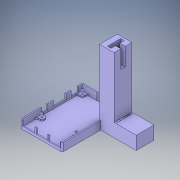
# Autodesk Inventor part: BaseStation.0027
Saved by Autodesk Inventor 2018 (Build 220112000, 112)
## iProperties
Material: Générique
Document SubType Name: Modeling
Density: 1 g/cm^3
Appearance: Par défaut(1)
Autodesk Inventor part; units mm, degrees
ref_plane "YZ Plane" through (0, 0, 0) normal (1, 0, 0) x (0, 1, 0)
ref_plane "XZ Plane" through (0, 0, 0) normal (0, 1, 0) x (-1, 0, 0)
ref_plane "XY Plane" through (0, 0, 0) normal (0, 0, 1) x (1, 0, 0)
sketch "Esquisse1" plane through (0, 0, 0) normal (0, 0, 1) x (1, 0, 0)
  line L0 (-30, -44.5) -> (30, -44.5)
  line L1 (30, -44.5) -> (30, 44.5)
  line L2 (30, 44.5) -> (-30, 44.5)
  line L3 (-30, 44.5) -> (-30, -44.5)
  line L4 (-30, -44.5) -> (30, 44.5) construction
  line L5 (30, -44.5) -> (-30, 44.5) construction
  point P0 (0, 0)
  dimension "Largeur_boite" = 60
  dimension "Longueur_boite" = 89
  constraints: 12 end point, 2 midpoint, 2 parallel, 1 horizontal, 1 perpendicular
  measures "Largeur_boite" distance of L2.end L1.end
  measures "Longueur_boite" distance of L1.end L0.end
extrude "Embase" add sketch "Esquisse1" along normal mid plane 11.5
shell "Coque" thickness 1.6 removed faces 1 at (-10, 14.8333, 5.75)
sketch "Esquisse2" plane through (-28.4, -42.9, -4.15) normal (0, 0, 1) x (1, 0, 0)
  line L0 (0, 85.8) -> (7.5, 85.8)
  line L1 (7.5, 85.8) -> (7.5, 78.3)
  line L2 (7.5, 78.3) -> (0, 78.3)
  line L3 (0, 78.3) -> (0, 85.8)
  line L4 (0, 85.8) -> (7.5, 78.3) construction
  line L5 (7.5, 85.8) -> (0, 78.3) construction
  line L6 (0, 27.8) -> (7.5, 27.8)
  line L7 (7.5, 27.8) -> (7.5, 20.3)
  line L8 (7.5, 20.3) -> (0, 20.3)
  line L9 (0, 20.3) -> (0, 27.8)
  line L10 (0, 27.8) -> (7.5, 20.3) construction
  line L11 (7.5, 27.8) -> (0, 20.3) construction
  line L12 (49.3, 85.8) -> (56.8, 85.8)
  line L13 (56.8, 85.8) -> (56.8, 78.3)
  line L14 (56.8, 78.3) -> (49.3, 78.3)
  line L15 (49.3, 78.3) -> (49.3, 85.8)
  line L16 (49.3, 85.8) -> (56.8, 78.3) construction
  line L17 (56.8, 85.8) -> (49.3, 78.3) construction
  line L18 (48.7, 27.8) -> (56.8, 27.8)
  line L19 (56.8, 27.8) -> (56.8, 20.3)
  line L20 (56.8, 20.3) -> (48.7, 20.3)
  line L21 (48.7, 20.3) -> (48.7, 27.8)
  line L22 (48.7, 27.8) -> (56.8, 20.3) construction
  line L23 (56.8, 27.8) -> (48.7, 20.3) construction
  line L24 (0, 85.8) -> (56.8, 85.8) projected
  line L25 (0, 0) -> (0, 85.8) projected
  line L26 (56.8, 85.8) -> (56.8, 0) projected
  point P0 (28.4, 42.9)
  point P1 (3.75, 82.05)
  point P2 (3.75, 24.05)
  point P3 (53.05, 82.05)
  point P4 (52.75, 24.05)
  point P5 (3.75, 24.05)
  point P6 (52.75, 24.05)
  point P7 (53.05, 82.05)
  point P8 (3.75, 82.05)
  dimension "d5" = 58
  dimension "d6" = 49
  dimension "Largeur_support" = 7.5
  dimension "d8" = 7.5
  dimension "d9" = 7.5
  dimension "d10" = 7.5
  constraints: 48 end point, 12 midpoint, 8 parallel, 5 collinear, 4 horizontal, 4 perpendicular, 4 point on line, 2 horizontal alignment
  measures "d5" vertical distance of point (53.05, 82.05) point (52.75, 24.05)
  measures "d6" distance of point (52.75, 24.05) point (3.75, 24.05)
  measures "Largeur_support" distance of L0.end L1.end
  measures "d8" distance of L1.end L2.end
  measures "d9" distance of L13.end L14.end
  measures "d10" distance between parallel lines of L8 L6
extrude "Support axe" add sketch "Esquisse2" along normal blind 2
sketch "Esquisse3" plane through (-28.4, -42.9, -2.15) normal (0, 0, 1) x (1, 0, 0)
  line L0 (49.3, 85.8) -> (56.8, 85.8) construction
  line L1 (49.3, 85.8) -> (49.3, 78.3) construction
  line L2 (49.3, 78.3) -> (56.8, 78.3) construction
  line L3 (56.8, 85.8) -> (56.8, 78.3) construction
  line L4 (0, 85.8) -> (7.5, 85.8) construction
  line L5 (0, 78.3) -> (0, 85.8) construction
  line L6 (0, 78.3) -> (7.5, 78.3) construction
  line L7 (7.5, 78.3) -> (7.5, 85.8) construction
  line L8 (7.5, 27.8) -> (0, 27.8) construction
  line L9 (0, 20.3) -> (0, 27.8) construction
  line L10 (0, 20.3) -> (7.5, 20.3) construction
  line L11 (7.5, 20.3) -> (7.5, 27.8) construction
  line L12 (56.8, 27.8) -> (48.7, 27.8) construction
  line L13 (48.7, 27.8) -> (48.7, 20.3) construction
  line L14 (48.7, 20.3) -> (56.8, 20.3) construction
  line L15 (56.8, 27.8) -> (56.8, 20.3) construction
  circle A0 centre (3.75, 82.05) radius 1.25
  circle A1 centre (52.75, 82.05) radius 1.25
  circle A2 centre (52.75, 24.05) radius 1.25
  circle A3 centre (3.75, 24.05) radius 1.25
  point P0 (28.4, 42.9)
  point P1 (7.5, 24.05)
  point P2 (48.7, 24.05)
  point P3 (7.5, 82.05)
  point P4 (49.3, 82.05)
  point P5 (3.75, 78.3)
  point P6 (53.05, 78.3)
  point P7 (3.75, 20.3)
  point P8 (52.75, 20.3)
  dimension "Hauteur_axe" = 2.5
  dimension "d14" = 2.5
  dimension "d15" = 2.5
  dimension "d16" = 2.5
  dimension "d54" = 3.45
  constraints: 8 midpoint, 4 centre point, 4 horizontal alignment, 3 vertical alignment
  measures "Hauteur_axe" diameter of A0
  measures "d14" diameter of A1
  measures "d15" diameter of A3
  measures "d16" diameter of A2
  measures "d54" distance from line of L1 A1.centre
extrude "Axe" add sketch "Esquisse3" along normal blind 7
sketch "Esquisse4" plane through (-30, -44.5, -5.75) normal (0, -1, 0) x (1, 0, 0)
  line L0 (3.5, 4) -> (21, 4)
  line L1 (21, 4) -> (21, 11.5)
  line L2 (21, 11.5) -> (3.5, 11.5)
  line L3 (3.5, 11.5) -> (3.5, 4)
  line L4 (23, 4) -> (39, 4)
  line L5 (39, 4) -> (39, 11.5)
  line L6 (39, 11.5) -> (23, 11.5)
  line L7 (23, 11.5) -> (23, 4)
  line L8 (41, 4) -> (57, 4)
  line L9 (57, 4) -> (57, 11.5)
  line L10 (57, 11.5) -> (41, 11.5)
  line L11 (41, 11.5) -> (41, 4)
  line L12 (0, 11.5) -> (0, 0) projected
  line L13 (0, 11.5) -> (60, 11.5) projected
  line L14 (60, 0) -> (0, 0) projected
  point P0 (30, 5.75)
  dimension "d19" = 17.5
  dimension "d20" = 16
  dimension "d21" = 16
  dimension "d22" = 3.5
  dimension "d23" = 2
  dimension "d24" = 2
  dimension "d28" = 4
  constraints: 24 end point, 6 parallel, 3 collinear, 3 horizontal, 3 perpendicular, 2 point on line
  measures "d19" distance of L1.end L2.end
  measures "d20" distance of L5.end L6.end
  measures "d21" distance of L9.end L10.end
  measures "d22" distance between parallel lines of L12 L3
  measures "d23" distance between parallel lines of L1 L7
  measures "d24" distance between parallel lines of L5 L11
  measures "d28" distance between parallel lines of L14 L0
extrude "Passage USB/Ethernet" cut sketch "Esquisse4" against normal up to surface (1.6 mm away)
sketch "Esquisse6" plane through (-30, -44.5, 5.75) normal (-1, 0, 0) x (0, 0, 1)
  line L0 (-7, 64) -> (0, 64)
  line L1 (0, 64) -> (0, 46)
  line L2 (0, 46) -> (-7, 46)
  line L3 (-7, 46) -> (-7, 64)
  line L4 (-11.5, 89) -> (0, 89) projected
  line L5 (0, 89) -> (0, 0) projected
  point P0 (-5.75, 44.5)
  dimension "d29" = 25
  dimension "d30" = 18
  dimension "profondeur_passage" = 7
  constraints: 8 end point, 2 parallel, 1 collinear, 1 horizontal, 1 perpendicular
  measures "d29" distance between parallel lines of L4 L0
  measures "d30" distance of L0.end L1.end
  measures "profondeur_passage" distance between parallel lines of L5 L3
extrude "Passage HDMI" cut sketch "Esquisse6" against normal up to surface (1.6 mm away)
sketch "Esquisse8" plane through (-30, -44.5, -5.75) normal (-1, 0, 0) x (0, 0, 1)
  line L0 (4.5, 81.5) -> (11.5, 81.5)
  line L1 (11.5, 81.5) -> (11.5, 71.5)
  line L2 (11.5, 71.5) -> (4.5, 71.5)
  line L3 (4.5, 71.5) -> (4.5, 81.5)
  line L4 (11.5, 89) -> (11.5, 64) projected
  line L5 (0, 89) -> (11.5, 89) projected
  point P0 (5.75, 44.5)
  dimension "d34" = 10
  dimension "d35" = 7
  dimension "d36" = 7.5
  constraints: 8 end point, 2 parallel, 1 collinear, 1 horizontal, 1 perpendicular
  measures "d34" distance of L0.end L1.end
  measures "d35" distance between parallel lines of L4 L3
  measures "d36" distance between parallel lines of L5 L0
extrude "Passage chargeur" cut sketch "Esquisse8" against normal up to surface (1.6 mm away)
sketch "Esquisse10" plane through (-30, 44.5, 5.75) normal (0, 1, 0) x (1, 0, 0)
  line L0 (37.5, 11.5) -> (22.5, 11.5)
  line L1 (22.5, 11.5) -> (22.5, 0)
  line L2 (22.5, 0) -> (37.5, 0)
  line L3 (37.5, 0) -> (37.5, 11.5)
  line L4 (37.5, 11.5) -> (22.5, 0) construction
  line L5 (22.5, 11.5) -> (37.5, 0) construction
  line L6 (60, 0) -> (0, 0) projected
  point P0 (30, 5.75)
  dimension "d39" = 15
  constraints: 12 end point, 2 midpoint, 2 parallel, 1 collinear, 1 horizontal, 1 perpendicular
  measures "d39" distance of L1.end L2.end
extrude "Passage SD" cut sketch "Esquisse10" against normal up to surface (1.6 mm away)
sketch "Esquisse11" plane through (-30, -44.5, -5.75) normal (-1, 0, 0) x (0, 0, 1)
  line L0 (4.5, 37.75) -> (11.5, 37.75)
  line L1 (11.5, 37.75) -> (11.5, 29.25)
  line L2 (11.5, 29.25) -> (4.5, 29.25)
  line L3 (4.5, 29.25) -> (4.5, 37.75)
  line L4 (0, 89) -> (11.5, 89) projected
  line L5 (11.5, 46) -> (11.5, 0) projected
  point P0 (5.75, 44.5)
  dimension "d42" = 51.25
  dimension "d43" = 8.5
  dimension "d44" = 7
  constraints: 8 end point, 2 parallel, 1 collinear, 1 horizontal, 1 perpendicular
  measures "d42" distance between parallel lines of L4 L0
  measures "d43" distance of L0.end L1.end
  measures "d44" distance between parallel lines of L5 L3
extrude "Passage Jack" cut sketch "Esquisse11" against normal up to surface (1.6 mm away)
chamfer "Chanfrein entrée sur axe" distance 0.3 angle 45 4 edges at (-25.9, 39.15, 4.85) (23.1, 39.15, 4.85) (23.1, -18.85, 4.85) (-25.9, -18.85, 4.85)
fillet "Congé coins" radius 2 4 edges at (-30, 44.5, 0) (30, 44.5, 0) (30, -44.5, 0) (-30, -44.5, 0)
fillet "Congé support axe" radius 2.5 14 edges at (-28.4, -22.6, -3.15) (-20.9, -22.6, -3.15) (-20.9, -15.1, -3.15) (-28.4, -15.1, -3.15) (-28.4, 35.4, -3.15) (-20.9, 35.4, -3.15) (-20.9, 42.9, -3.15) (20.9, 42.9, -3.15) (20.9, 35.4, -3.15) (28.4, 35.4, -3.15) (28.4, -22.6, -3.15) (20.3, -22.6, -3.15) (20.3, -15.1, -3.15) (28.4, -15.1, -3.15)
sketch "Sketch14" plane through (30, -42.5, -5.75) normal (1, 0, 0) x (0, 0, -1)
  line L0 (0, 53.25) -> (-105.41, 53.25)
  line L1 (-105.41, 53.25) -> (-105.41, 78.65)
  line L2 (-105.41, 78.65) -> (0, 78.65)
  line L3 (0, 78.65) -> (0, 53.25)
  line L4 (0, 85) -> (-11.5, 85) projected
  line L5 (0, 85) -> (0, 0) projected
  point P0 (-5.75, 42.5)
  dimension "d59" = 105.41
  dimension "d60" = 25.4
  dimension "d61" = 6.35
  constraints: 8 end point, 2 parallel, 1 collinear, 1 horizontal, 1 perpendicular
  measures "d59" distance of L1.end L2.end
  measures "d60" distance of L0.end L1.end
  measures "d61" distance between parallel lines of L4 L2
extrude "Extrusion9" add sketch "Sketch14" along normal blind 19.05 and the other way blind 1.6
sketch "Sketch15" plane through (28.4, 10.75, 99.66) normal (0, 0, 1) x (1, 0, 0)
  line L0 (20.65, 3.175) -> (7.95, 3.175)
  line L1 (7.95, 3.175) -> (7.95, 22.225)
  line L2 (7.95, 22.225) -> (20.65, 22.225)
  line L3 (20.65, 22.225) -> (20.65, 3.175)
  line L4 (20.65, 0) -> (0, 0) projected
  line L5 (20.65, 25.4) -> (20.65, 0) projected
  line L6 (13.03, 3.175) -> (13.03, 22.225)
  line L7 (7.95, 3.175) -> (7.95, 22.225)
  line L8 (13.03, 9.525) -> (20.65, 9.525)
  line L9 (20.65, 0) -> (20.65, 25.4) projected
  line L10 (13.03, 15.875) -> (20.65, 15.875)
  point P0 (-28.4, -10.75)
  dimension "d66" = 12.7
  dimension "d67" = 19.05
  dimension "d68" = 3.175
  dimension "d69" = 5.08
  dimension "d70" = 6.35
  dimension "d71" = 9.525
  constraints: 16 end point, 8 point on line, 4 parallel, 2 collinear, 2 horizontal, 2 perpendicular
  measures "d66" distance of L1.end L2.end
  measures "d67" distance of L0.end L1.end
  measures "d68" distance between parallel lines of L4 L0
  measures "d69" distance between parallel lines of L6 L7
  measures "d70" distance between parallel lines of L10 L8
  measures "d71" distance between parallel lines of L4 L8
extrude "Extrusion10" cut sketch "Sketch15" against normal blind 25.4 contours L0 L1 L2 L6 | L8 L6 L10 L3
sketch "Sketch17" plane through (0, 0, -5.75) normal (0, 0, -1) x (-1, 0, 0)
  line L0 (-49.05, 36.15) -> (-28.4, 36.15) projected
  line L1 (-49.05, 36.15) -> (-80.8, 36.15)
  line L2 (-80.8, 36.15) -> (-80.8, 10.75)
  line L3 (-80.8, 10.75) -> (-49.05, 10.75)
  line L4 (-49.05, 10.75) -> (-49.05, 36.15)
  line L5 (-30, 10.75) -> (-49.05, 10.75) projected
  point P0 (0, 0)
  dimension "d74" = 31.75
  constraints: 8 end point, 2 parallel, 1 collinear, 1 horizontal, 1 perpendicular
  measures "d74" distance between parallel lines of L4 L2
extrude "Extrusion11" add sketch "Sketch17" against normal blind 19.05
sketch "Sketch18" plane through (0, 0, 13.3) normal (0, 0, 1) x (1, 0, 0)
  line L0 (51.59, 13.29) -> (49.05, 13.29)
  line L1 (49.05, 13.29) -> (49.05, 33.61)
  line L2 (49.05, 33.61) -> (51.59, 33.61)
  line L3 (51.59, 33.61) -> (51.59, 13.29)
  line L4 (49.05, 10.75) -> (49.05, 36.15) projected
  line L5 (49.05, 10.75) -> (80.8, 10.75) projected
  point P0 (0, 0)
  dimension "d77" = 2.54
  dimension "d78" = 20.32
  dimension "d79" = 2.54
  constraints: 8 end point, 2 parallel, 1 collinear, 1 horizontal, 1 perpendicular
  measures "d77" distance of L1.end L2.end
  measures "d78" distance of L0.end L1.end
  measures "d79" distance between parallel lines of L5 L0
extrude "Extrusion12" cut sketch "Sketch18" against normal blind 15.875
sketch "Sketch19" plane through (49.05, -42.5, -5.75) normal (1, 0, 0) x (0, 0, -1)
  line L0 (-19.05, 55.79) -> (-3.175, 55.79)
  line L1 (-3.175, 55.79) -> (-3.175, 76.11)
  line L2 (-3.175, 76.11) -> (-19.05, 76.11)
  line L3 (-19.05, 76.11) -> (-19.05, 55.79)
  line L4 (-19.05, 76.11) -> (-3.175, 76.11) projected
  line L5 (-19.05, 55.79) -> (-3.175, 55.79) projected
  line L6 (-3.175, 55.79) -> (-3.175, 76.11) projected
  point P0 (-5.75, 42.5)
  dimension "d82" = 15.875
  constraints: 8 end point, 3 collinear, 2 parallel, 1 horizontal, 1 perpendicular
  measures "d82" distance between parallel lines of L1 L3
extrude "Extrusion13" cut sketch "Sketch19" against normal blind 20.6502
equation "\"d8\" = Largeur_support"
equation "\"d9\" = Largeur_support"
equation "\"d10\" = Largeur_support"
equation "\"d14\" = Hauteur_axe"
equation "\"d15\" = Hauteur_axe"
equation "\"d16\" = d14"
equation "\"d35\" = profondeur_passage"
equation "\"d44\" = profondeur_passage"
